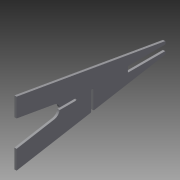
# Autodesk Inventor part: stand
Saved by Autodesk Inventor 2017 (Build 210142000, 142)
## iProperties
Created: 2019-02-02
Part Number: stand
Material: Generic
Document SubType Name: Modeling
Designer: ari
Density: 1 g/cm^3
Appearance: Default
Author: ari
Autodesk Inventor part; units mm, degrees
ref_plane "YZ Plane" through (0, 0, 0) normal (1, 0, 0) x (0, 1, 0)
ref_plane "XZ Plane" through (0, 0, 0) normal (0, 1, 0) x (-1, 0, 0)
ref_plane "XY Plane" through (0, 0, 0) normal (0, 0, 1) x (1, 0, 0)
sketch "Sketch1" plane through (0, 0, 0) normal (1, 0, 0) x (0, 1, 0)
  line L0 (0, 0) -> (237, -41.7895)
  line L1 (237, -41.7895) -> (237, -46.4413)
  line L2 (237, -60.0931) -> (0, -101.8825)
  line L3 (0, -101.8825) -> (0, -71.8825)
  line L4 (0, -71.8825) -> (68.5, -59.8042)
  line L5 (68.5, -59.8042) -> (68.5, -42.0784)
  line L6 (68.5, -42.0784) -> (0, -30)
  line L7 (0, -30) -> (0, 0)
  line L8 (122.05, -80.3618) -> (122.05, -50.9413)
  line L9 (177, -50.9413) -> (68.5, -50.9413) construction
  line L10 (237, -46.4413) -> (177, -46.4413)
  line L11 (177, -46.4413) -> (177, -55.4413)
  line L12 (177, -55.4413) -> (237, -55.4413)
  line L13 (237, -55.4413) -> (237, -46.4413) construction
  line L14 (237, -46.4413) -> (237, -55.4413) construction
  line L15 (237, -55.4413) -> (237, -60.0931)
  line L16 (122.05, -50.9413) -> (118.5, -50.9413)
  line L17 (118.5, -50.9413) -> (118.5, -80.9878)
  line L18 (-47.4, 0) -> (284.4, 0) construction
  line L19 (68.5, -49.1663) -> (93.5, -49.1663)
  line L20 (93.5, -49.1663) -> (93.5, -52.7163)
  line L21 (93.5, -52.7163) -> (68.5, -52.7163)
  line L22 (68.5, -52.7163) -> (68.5, -49.1663)
  arc A0 (93.5, -52.7163) -> (93.5, -49.1663) centre (93.5, -50.9413) ccw
  arc A1 (122.05, -50.9413) -> (118.5, -50.9413) centre (120.275, -50.9413) ccw
  dimension "d1" = 3.55
  dimension "d2" = 9
  dimension "d3" = 60
  dimension "d4" = 177
  dimension "d5" = 30
  dimension "d7" = 10
  dimension "d9" = 15
  dimension "d10" = 101.8825
  dimension "d11" = 237
  dimension "d12" = 50
  dimension "d13" = 25
  dimension "d14" = 3.55
  constraints: 44 end point, 12 parallel, 5 midpoint, 5 point on line, 4 point on circle, 4 vertical, 3 horizontal, 2 centre point, 2 collinear, 2 perpendicular, 3 other
  measures "d1" distance of L8.end L16.end
  measures "d2" distance between parallel lines of L12 L10
  measures "d3" distance of L11.end L12.end
  measures "d4" distance between parallel lines of L7 L11
  measures "d5" distance of L6.end L0.start
  measures "d7" angle of L0 L18
  measures "d9" distance from line of L0 L10.end
  measures "d10" distance of L2.end L0.start
  measures "d11" horizontal distance of L0.end L0.start
  measures "d12" distance between parallel lines of L5 L17
  measures "d13" distance of L19.start L19.end
  measures "d14" distance of L19.end L20.end
extrude "Extrusion1" add sketch "Sketch1" along normal blind 3.5 contours L0 L1 L10 L11 L12 L15 L2 L8 A1 L17 L3 L4 L5 L21 A0 L19 L6 L7
fillet "Fillet1" radius 10 2 edges at (1.75, 68.5, -42.0784) (1.75, 68.5, -59.8042)
fillet "Fillet1" radius 1 8 edges at (1.75, 177, -46.4413) (1.75, 177, -55.4413) (1.75, 122.05, -80.3618) (1.75, 118.5, -80.9878) (1.75, 237, -41.7895) (1.75, 237, -46.4413) (1.75, 237, -55.4413) (1.75, 237, -60.0931)
equation "\"d1\" = d + u"
equation "\"d14\" = d + u"
equation "\"d15\" = d"
equation "\"d\" = 3.5"
equation "\"u\" = 0.05"
body "Solid1"
